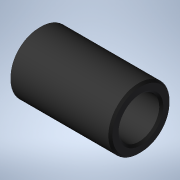
# Autodesk Inventor part: C-KNCLA4-6-10
Saved by Autodesk Inventor 2021 (Build 250183000, 183)
## iProperties
Created: 2025-01-07
Part Number: C-KNCLA4-6-10
Material: Generic
Catalog Web Link: www.cadenas.de
Description: C-KNCLA-Economy Metal Collars Standard
Vendor: MISUMI
Document SubType Name: Modeling
Designer: psAdmin
Manufacturer: MISUMI
Mass: 0.155823 g
Surface Area: 3.38214 cm^2
Volume: 0.155823 cm^3
Density: 1 g/cm^3
Appearance: PSOLRGB-175-175-175
Category: PARTsolutions
Company: MISUMI
Title: C-KNCLA4-6-10
Author: Cadenas PARTsolutions
Comments: Economy Metal Collars Standard
PSOL_IDENT_0: {$CADENAS_DATA/23d-libs/misumi/metric/26_washers_collars/c_kncla.prj},173 {VTYP=3D},{NB=C-KNCLA4-6-1
PSOL_IDENT_1: 0},{LINA=C-KNCLA4-6-10},{NN=C-KNCLA},{DATE=16.11.2023 12:01:01},{GEOMDATE=13.11.2023 13:21:43},{VERS
PSOL_IDENT_2: ION=},{LINEID=20},{WBVAR=D,L},{WBNUMERIC=D,L}  {NB=C-KNCLA4-6-10},{LINA=C-KNCLA4-6-10},{KT=DUMMY},{P
PSOL_IDENT_3: N=C-KNCLA4-6-10},{TYPE=C-KNCLA},{V=4},{D=6},{D1=6,8,10},{L=10},{LALG=10,12,15},{C=0.2}
NB: C-KNCLA4-6-10
NN: C-KNCLA
NT: Economy Metal Collars Standard
NBSYN: $PN.
LINA: C-KNCLA4-6-10
CATALOG: Misumi
PN: C-KNCLA4-6-10
V: 4
D: 6
L: 10
SUPPLIER: MISUMI
ARTICLENO: C-KNCLA4-6-10
BOMINFO: C-KNCLA4-6-10
CREATOR: CADENAS GmbH
Autodesk Inventor part; units mm, degrees
ref_plane "YZ Plane" through (0, 0, 0) normal (1, 0, 0) x (0, 1, 0)
ref_plane "XZ Plane" through (0, 0, 0) normal (0, 1, 0) x (-1, 0, 0)
ref_plane "XY Plane" through (0, 0, 0) normal (0, 0, 1) x (1, 0, 0)
sketch "_____1" plane through (0, 0, 0) normal (0, 0, 1) x (1, 0, 0)
  line L0 (10, 0) -> (0, 0)
  line L1 (0, 0) -> (0, 2.8)
  line L2 (0, 2.8) -> (0.2, 3)
  line L3 (0.2, 3) -> (9.8, 3)
  line L4 (9.8, 3) -> (10, 2.8)
  line L5 (10, 2.8) -> (10, 0)
  line L6 (10, 0) -> (0, 0)
  constraints: 14 end point
revolve "Revolution1" add sketch "_____1" angle 360 about axis through (10, 0, 0) along (1, 0, 0)
sketch "_____2" plane through (0, 0, 0) normal (0, 0, 1) x (1, 0, 0)
  line L0 (20, 0) -> (-20, 0)
  line L1 (0, 0) -> (0, 2.2)
  line L2 (0, 2.2) -> (0.2, 2)
  line L3 (0.2, 2) -> (9.8, 2)
  line L4 (9.8, 2) -> (10, 2.2)
  line L5 (10, 2.2) -> (10, 0)
  line L6 (10, 0) -> (0, 0)
  constraints: 14 end point
revolve "Revolution2" cut sketch "_____2" angle 360 about axis through (20, 0, 0) along (1, 0, 0)
body "Solid1"
